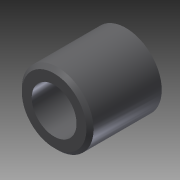
# Autodesk Inventor part: D-040
Saved by Autodesk Inventor 2015 (Build 190159000, 159)
## iProperties
Company: MARCHA TECHNOLOGY
Created: 2013-10-28
Part Number: D-040
Document SubType Name: Modeling
Designer: O.Martin
Density: 1 g/cm^3
Project: WITBOXprinter_v04
Description: CASQUILLO CONICO RACOR
Stock Number: 28656
Material: Generic
Appearance: Gray
Author: O.Martin
Autodesk Inventor part; units mm, degrees
ref_plane "YZ Plane" through (0, 0, 0) normal (1, 0, 0) x (0, 1, 0)
ref_plane "XZ Plane" through (0, 0, 0) normal (0, 1, 0) x (-1, 0, 0)
ref_plane "XY Plane" through (0, 0, 0) normal (0, 0, 1) x (1, 0, 0)
sketch "Boceto1" plane through (0, 0, 0) normal (0, 0, 1) x (1, 0, 0)
  line L0 (0, 4) -> (0, 0)
  line L1 (-2, 4) -> (-2, 0)
  line L2 (-2, 0) -> (-1.25, 0)
  line L3 (-1.25, 0) -> (-1.25, 2.701)
  line L4 (-1.25, 2.701) -> (-2, 4)
  dimension "d0" = 4
  dimension "d1" = 2.5
  dimension "d2" = 4
  dimension "d3" = 30
  constraints: 10 end point, 2 perpendicular, 1 coincident, 1 horizontal alignment, 1 parallel, 1 vertical
  measures "d0" diameter of L1 L0
  measures "d1" diameter of L3 L0
  measures "d2" distance of L1.start L1.end
  measures "d3" angle of L3 L4
revolve "Revolución1" add sketch "Boceto1" angle 360 about axis through (0, 4, 0) along (0, -1, 0)
chamfer "Chaflán1" distance 0.2 angle 45 1 edges at (2, 0, 0)
body "Solid1"
